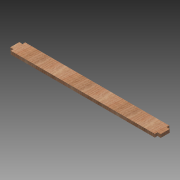
# Autodesk Inventor part: viga diagonal
Saved by Autodesk Inventor 2015 (Build 190159000, 159)
## iProperties
Created: 2016-02-08
Part Number: viga diagonal
Material: Wood (Birch)
Document SubType Name: Modeling
Designer: iberopuebla
Density: 0.55 g/cm^3
Appearance: Birch - Natural Polished
Author: iberopuebla
Autodesk Inventor part; units mm, degrees
ref_plane "YZ Plane" through (0, 0, 0) normal (1, 0, 0) x (0, 1, 0)
ref_plane "XZ Plane" through (0, 0, 0) normal (0, 1, 0) x (-1, 0, 0)
ref_plane "XY Plane" through (0, 0, 0) normal (0, 0, 1) x (1, 0, 0)
sketch "Sketch1" plane through (0, 0, 0) normal (0, 0, 1) x (1, 0, 0)
  line L0 (1035.4474, -2.1782) -> (1835.4474, -2.1782)
  line L1 (1835.4474, -82.1782) -> (1035.4474, -82.1782)
  line L2 (1035.4474, -17.1782) -> (1017.4474, -17.1782)
  line L3 (1017.4474, -17.1782) -> (1017.4474, -67.1782)
  line L4 (1017.4474, -67.1782) -> (1035.4474, -67.1782)
  line L5 (1835.4474, -17.1782) -> (1853.4474, -17.1782)
  line L6 (1853.4474, -17.1782) -> (1853.4474, -67.1782)
  line L7 (1853.4474, -67.1782) -> (1835.4474, -67.1782)
  line L8 (1835.4474, -2.1782) -> (1835.4474, -17.1782)
  line L9 (1835.4474, -67.1782) -> (1835.4474, -82.1782)
  line L10 (1035.4474, -82.1782) -> (1035.4474, -67.1782)
  line L11 (1035.4474, -17.1782) -> (1035.4474, -2.1782)
  point P0 (0, 0)
  dimension "d10" = 800
  dimension "d11" = 80
  dimension "d12" = 50
  dimension "d13" = 18
  dimension "d14" = 50
  dimension "d15" = 18
  dimension "d19" = 15
  dimension "d20" = 800
  dimension "d21" = 18
  constraints: 24 end point, 7 parallel, 4 perpendicular, 3 horizontal, 1 point on line
  measures "d10" distance of L0.start L0.end
  measures "d11" distance between parallel lines of L1 L0
  measures "d12" distance of L2.end L3.end
  measures "d13" distance of L2.start L2.end
  measures "d14" distance of L5.end L6.end
  measures "d15" distance of L6.end L7.end
  measures "d19" distance between parallel lines of L2 L0
  measures "d20" distance of L1.start L1.end
  measures "d21" distance between parallel lines of L10 L3
extrude "Extrusion1" add sketch "Sketch1" along normal blind 18
sketch "Sketch2" plane through (0, 0, 18) normal (0, 0, 1) x (1, 0, 0)
  line L0 (1035.4474, -17.1782) -> (1034.3161, -16.0469)
  line L1 (1035.4474, -17.1782) -> (1037.0474, -17.1782) construction
  line L2 (1035.4474, -67.1782) -> (1034.3161, -68.3096)
  line L3 (1835.4474, -17.1782) -> (1836.5788, -16.0469)
  line L4 (1835.4474, -67.1782) -> (1836.5788, -68.3096)
  circle A0 centre (1836.5788, -68.3096) radius 1.6
  circle A1 centre (1836.5788, -16.0469) radius 1.6
  circle A2 centre (1034.3161, -68.3096) radius 1.6
  circle A3 centre (1034.3161, -16.0469) radius 1.6
  point P0 (0, 0)
  dimension "d22" = 1.6
  dimension "d23" = 135
  dimension "d24" = 3.2
  dimension "d25" = 3.2
  dimension "d26" = 3.2
  dimension "d27" = 3.2
  constraints: 10 end point, 4 centre point, 3 coincident, 2 perpendicular, 1 equal length, 1 horizontal, 1 parallel, 1 point on line
  measures "d22" distance of L0.start L0.end
  measures "d23" angle of L1 L0
  measures "d24" diameter of A0
  measures "d25" diameter of A1
  measures "d26" diameter of A2
  measures "d27" diameter of A3
extrude "Extrusion2" cut sketch "Sketch2" against normal blind 20
body "Solid1"
